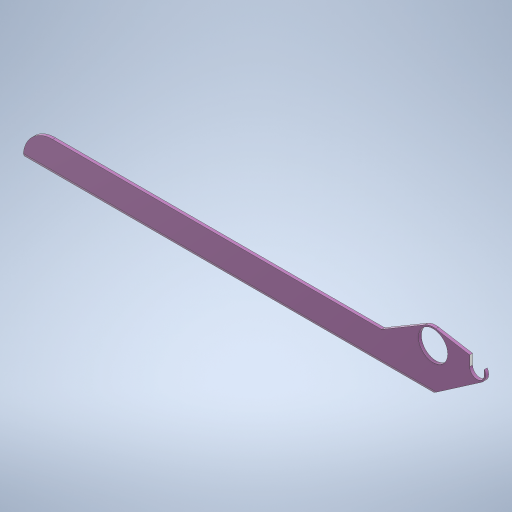
# Autodesk Inventor part: hoja de filo
Saved by Autodesk Inventor 2023 (Build 270158030, 158C)
## iProperties
Created: 2022-05-25
Part Number: hoja de filo
Material: Genérico
Document SubType Name: Modeling
Designer: isaac
Density: 1 g/cm^3
Appearance: Valor por defecto
Author: isaac
Autodesk Inventor part; units mm, degrees
ref_plane "YZ Plane" through (0, 0, 0) normal (1, 0, 0) x (0, 1, 0)
ref_plane "XZ Plane" through (0, 0, 0) normal (0, 1, 0) x (-1, 0, 0)
ref_plane "XY Plane" through (0, 0, 0) normal (0, 0, 1) x (1, 0, 0)
sketch "Boceto4" plane through (0, 0, 0) normal (0, 0, 1) x (1, 0, 0)
  circle A0 centre (0, 140) radius 50
  circle A1 centre (150, 140) radius 25
  arc A2 (167.0429, 115.3112) -> (155, 169.5804) centre (150, 140) ccw
  arc A3 (9.1667, 194.2307) -> (-27.9698, 187.3571) centre (0, 140) ccw
  line L0 (155, 169.5804) -> (9.1667, 194.2307)
  line L1 (0, 0) -> (167.0429, 115.3112)
  line L2 (0, 0) -> (-1400, 0)
  line L3 (-27.9698, 187.3571) -> (-175.8786, 100)
  line L4 (-175.8786, 100) -> (-1300, 100)
  arc A4 (-1300, 100) -> (-1400, 0) centre (-1300, 0) ccw
  dimension "d24" = 100
  dimension "d25" = 50
  dimension "d26" = 150
  dimension "d27" = 5
  dimension "d28" = 5
  dimension "d29" = 140
  dimension "d30" = 1400
  dimension "d32" = 100
  dimension "d33" = 171.7797
  constraints: 10 end point, 6 point on circle, 5 centre point, 5 tangent, 2 horizontal, 1 horizontal alignment, 1 point on line, 1 vertical alignment
  measures "d24" diameter of A0
  measures "d25" diameter of A1
  measures "d26" distance of A1.centre A0.centre
  measures "d27" radial gap between concentric circles of A1 A2
  measures "d28" radial gap between concentric circles of A0 A3
  measures "d29" distance of L1.start A0.centre
  measures "d30" distance of L1.start L2.end
  measures "d32" distance between parallel lines of L2 L4
  measures "d33" distance of L3.start L3.end
extrude "Extrusión3" add sketch "Boceto4" along normal mid plane 10
sketch "Boceto5" plane through (0, 0, 0) normal (1, 0, 0) x (0, 1, 0)
  line L0 (12, -5.0363) -> (-1, -0.3047)
  line L1 (-1, -0.3047) -> (-1, -5.0363)
  line L2 (-1, -5.0363) -> (12, -5.0363)
  line L3 (12, 6.2463) -> (-1, 1.77)
  line L4 (-1, 1.77) -> (-1, 6.2463)
  line L5 (-1, 6.2463) -> (12, 6.2463)
  point P0 (0, 0)
  dimension "d36" = 1
  dimension "d37" = 13
  dimension "d38" = 13
  dimension "d39" = 70
  dimension "d40" = 71
  dimension "d41" = 0.3047
  dimension "d42" = 1.77
  constraints: 12 end point, 2 perpendicular, 2 point on line, 1 vertical
  measures "d36" distance from line of L4 point (0, 0)
  measures "d37" distance from line of L1 L0.start
  measures "d38" distance of L4.end L3.start
  measures "d39" angle of L1 L0
  measures "d40" angle of L4 L3
  measures "d41" vertical distance of L0.end point (0, 0)
  measures "d42" vertical distance of point (0, 0) L3.end
extrude "Extrusión4" cut sketch "Boceto5" along normal through all both and the other way through all
sketch "Boceto6" plane through (0, 0, 5) normal (0, 0, 1) x (1, 0, 0)
  circle A0 centre (150, 140) radius 25 construction
  line L0 (125, 140) -> (175, 140)
  line L1 (175, 140) -> (175, 182.8378)
  line L2 (175, 182.8378) -> (125, 182.8378)
  line L3 (125, 182.8378) -> (125, 140)
  point P0 (0, 0)
  dimension "d45" = 42.8378
  dimension "d46" = 50
  dimension "d47" = 0
  constraints: 8 end point, 2 parallel, 1 horizontal, 1 horizontal alignment, 1 perpendicular, 1 other
  measures "d45" distance between parallel lines of L0 L2
  measures "d46" distance between parallel lines of L3 L1
  measures "d47" distance from line of point (150, 140) L0
extrude "Extrusión5" cut sketch "Boceto6" against normal through all
